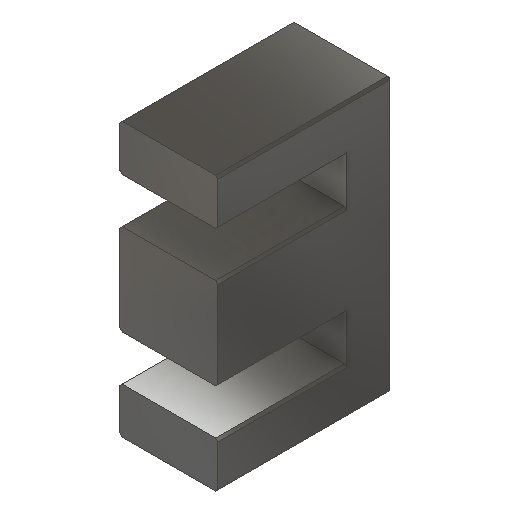
# Autodesk Inventor part: COTS_GENERIC_Transformer_Core
Saved by Autodesk Inventor 2026.1 (Build 301233000, 233)
## iProperties
Created: 2018-05-26
Part Number: COTS_GENERIC_Transformer_Core
Material: Stainless Steel
Document SubType Name: Modeling
Designer: Andrzej
Density: 8 g/cm^3
Appearance: Steel - Polished
Author: Andrzej
Autodesk Inventor part; units mm, degrees
ref_plane "YZ Plane" through (0, 0, 0) normal (1, 0, 0) x (0, 1, 0)
ref_plane "XZ Plane" through (0, 0, 0) normal (0, 1, 0) x (-1, 0, 0)
ref_plane "XY Plane" through (0, 0, 0) normal (0, 0, 1) x (1, 0, 0)
sketch "Sketch1" plane through (0, 0, 0) normal (0, 0, 1) x (1, 0, 0)
  line L0 (-10.8185, 29.4098) -> (2.1815, 29.4098)
  line L1 (2.1815, 29.4098) -> (2.1815, -6.8902)
  line L2 (2.1815, -6.8902) -> (-10.8185, -6.8902)
  line L3 (-10.8185, -6.8902) -> (-10.8185, 29.4098)
  point P0 (0, 0)
  dimension "d0" = 13
  dimension "d1" = 36.3
  constraints: 8 end point, 2 parallel, 1 horizontal, 1 perpendicular
  measures "d0" distance of L1.end L2.end
  measures "d1" distance of L0.end L1.end
extrude "Extrusion1" add sketch "Sketch1" along normal blind 6
sketch "Sketch2" plane through (0, 0, 6) normal (0, 0, 1) x (1, 0, 0)
  line L0 (2.1815, 29.4098) -> (-10.8185, 29.4098) projected
  line L1 (-10.8185, 29.4098) -> (-10.8185, -6.8902) projected
  line L2 (-10.8185, -6.8902) -> (2.1815, -6.8902) projected
  line L3 (2.1815, -6.8902) -> (2.1815, 29.4098) projected
  line L4 (2.1815, -0.7902) -> (-10.8185, -0.7902)
  line L5 (-10.8185, 29.4098) -> (-10.8185, -6.8902) projected
  line L6 (-10.8185, 5.2098) -> (2.1815, 5.2098)
  line L7 (2.1815, -6.8902) -> (2.1815, 29.4098) projected
  line L8 (-10.8185, 17.3098) -> (2.1815, 17.3098)
  line L9 (-10.8185, 23.3098) -> (2.1815, 23.3098)
  point P0 (0, 0)
  dimension "d4" = 6.1
  dimension "d5" = 6.1
  dimension "d6" = 12.1
  dimension "d7" = 12.1
  dimension "d8" = 36.3
  constraints: 8 end point, 8 point on line, 3 perpendicular, 1 horizontal
  measures "d4" distance between parallel lines of L2 L4
  measures "d5" distance between parallel lines of L0 L9
  measures "d6" distance between parallel lines of L8 L6
  measures "d7" distance between parallel lines of L2 L6
  measures "d8" distance of L2.end L0.start
extrude "Extrusion2" add sketch "Sketch2" along normal blind 17.1 contours L3 L9 L1 L0 | L3 L6 L1 L8 | L3 L2 L1 L4
chamfer "Chamfer1" distance 0.3 angle 45 16 edges at (-10.8185, 29.4098, 11.55) (-10.8185, 23.3098, 14.55) (-10.8185, 17.3098, 14.55) (2.1815, 17.3098, 14.55) (2.1815, 5.2098, 14.55) (-10.8185, 5.2098, 14.55) (-10.8185, -0.7902, 14.55) (2.1815, -0.7902, 14.55) (-10.8185, -6.8902, 11.55) (2.1815, -6.8902, 11.55) (2.1815, 29.4098, 11.55) (2.1815, 23.3098, 14.55) (-10.8185, 11.2598, 0) (2.1815, 11.2598, 0) (-4.3185, 29.4098, 0) (-4.3185, -6.8902, 0)
equation "\"d5\" = d4"
equation "\"d7\" = -0.5 * d6 + 0.5 * d8"
body "Solid1"
